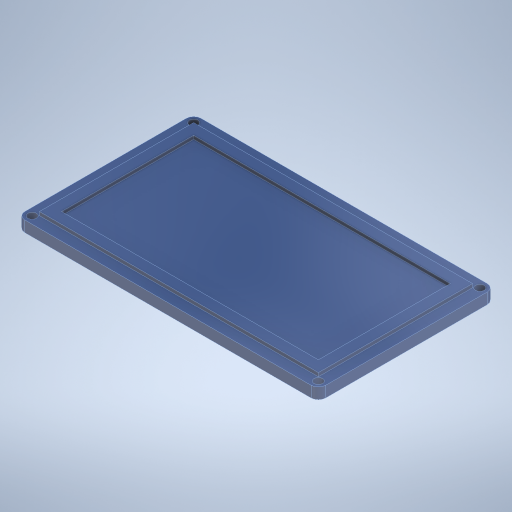
# Autodesk Inventor part: Tapa principal
Saved by Autodesk Inventor 2023 (Build 270158000, 158)
## iProperties
Created: 2023-03-20
Part Number: Tapa principal
Material: Plástico ABS
Document SubType Name: Modeling
Designer: sergi
Density: 1.06 g/cm^3
Appearance: Satinado con motas - Azul
Mass: 13.1603 g
Surface Area: 91.3712 cm^2
Volume: 12.4154 cm^3
Author: sergi
Autodesk Inventor part; units mm, degrees
ref_plane "YZ Plane" through (0, 0, 0) normal (1, 0, 0) x (0, 1, 0)
ref_plane "XZ Plane" through (0, 0, 0) normal (0, 1, 0) x (-1, 0, 0)
ref_plane "XY Plane" through (0, 0, 0) normal (0, 0, 1) x (1, 0, 0)
sketch "Boceto1" plane through (0, 0, 0) normal (0, 1, 0) x (-1, 0, 0)
  line L0 (-39, 24) -> (39, 24)
  line L1 (41, 22) -> (41, -22)
  line L2 (39, -24) -> (-39, -24)
  line L3 (-41, -22) -> (-41, 22)
  line L4 (-41, 24) -> (41, -24) construction
  line L5 (41, 24) -> (-41, -24) construction
  arc A0 (39, -24) -> (41, -22) centre (39, -22) ccw
  arc A1 (-41, -22) -> (-39, -24) centre (-39, -22) ccw
  arc A2 (-39, 24) -> (-41, 22) centre (-39, 22) ccw
  arc A3 (41, 22) -> (39, 24) centre (39, 22) ccw
  point P0 (0, 0)
  dimension "d0" = 82
  dimension "d1" = 48
  dimension "d2" = 2
  constraints: 12 end point, 8 point on circle, 8 point on line, 8 tangent, 4 centre point, 3 equal radius, 2 midpoint, 2 parallel, 1 horizontal, 1 perpendicular
  measures "d0" distance of L4.end L5.end
  measures "d1" distance of L5.start L4.end
  measures "d2" radius of A0
extrude "Extrusión1" add sketch "Boceto1" along normal blind 3
sketch "Boceto2" plane through (0, 3, 0) normal (0, 1, 0) x (1, 0, 0)
  line L0 (38, -21) -> (-38, -21)
  line L1 (-38, -21) -> (-38, 21)
  line L2 (-38, 21) -> (38, 21)
  line L3 (38, 21) -> (38, -21)
  line L4 (38, -21) -> (-38, 21) construction
  line L5 (-38, -21) -> (38, 21) construction
  line L6 (39, 24) -> (-39, 24) projected
  line L7 (41, -22) -> (41, 22) projected
  line L8 (35, -18) -> (-35, -18)
  line L9 (-35, -18) -> (-35, 18)
  line L10 (-35, 18) -> (35, 18)
  line L11 (35, 18) -> (35, -18)
  line L12 (35, -18) -> (-35, 18) construction
  line L13 (-35, -18) -> (35, 18) construction
  point P0 (0, 0)
  dimension "d5" = 3
  dimension "d6" = 3
  dimension "d7" = 3
  dimension "d8" = 3
  constraints: 24 end point, 4 midpoint, 4 parallel, 2 horizontal, 2 perpendicular
  measures "d5" distance between parallel lines of L6 L2
  measures "d6" distance between parallel lines of L7 L3
  measures "d7" distance between parallel lines of L3 L11
  measures "d8" distance between parallel lines of L2 L10
extrude "Extrusión2" add sketch "Boceto2" along normal blind 1
sketch "Boceto3" plane through (0, 0, 0) normal (0, -1, 0) x (1, 0, 0)
  point P0 (-39, 22)
hole "Agujero1" at (-39, 0, 22) direction (0, 1, 0) diameter 2.4 end through all
sketch "Boceto4" plane through (0, 0, 0) normal (0, -1, 0) x (1, 0, 0)
  point P0 (-39, -22)
hole "Agujero2" at (-39, 0, -22) direction (0, 1, 0) diameter 2.4 end through all
sketch "Boceto5" plane through (0, 0, 0) normal (0, -1, 0) x (1, 0, 0)
  point P0 (39, 22)
hole "Agujero3" at (39, 0, 22) direction (0, 1, 0) diameter 2.4 end through all
sketch "Boceto6" plane through (0, 0, 0) normal (0, -1, 0) x (1, 0, 0)
  point P0 (39, -22)
hole "Agujero4" at (39, 0, -22) direction (0, 1, 0) diameter 2.4 end through all
scale "Escala1" factors (2, 2, 2) then translate (0, 0, 0) bodies 1
